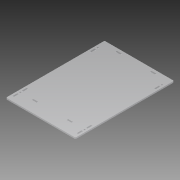
# Autodesk Inventor part: plastic_part_1
Saved by Autodesk Inventor 2013 (Build 170138000, 138)
## iProperties
Shininess: 20.0
Created: 2013-02-12
Part Number: plastic_part_1
Document SubType Name: Modeling
Designer: Noa Izumi
Material: Default
Density: 1 g/cm^3
Density: 0.0
Volumn: 0.0
Area: 0.0
PropertySet Name: Model Information
Control State: 0
Master: False
Checked Out: False
Author: Noa Izumi
Autodesk Inventor part; units mm, degrees
ref_plane "YZ Plane" through (0, 0, 0) normal (1, 0, 0) x (0, 1, 0)
ref_plane "XZ Plane" through (0, 0, 0) normal (0, 1, 0) x (-1, 0, 0)
ref_plane "XY Plane" through (0, 0, 0) normal (0, 0, 1) x (1, 0, 0)
sketch "Sketch1" plane through (0, 0, 0) normal (0, 0, 1) x (1, 0, 0)
  line L0 (0, 0) -> (148, 0)
  line L1 (148, 0) -> (148, 210)
  line L2 (148, 210) -> (0, 210)
  line L3 (0, 210) -> (0, 0)
  dimension "d0" = 148
  dimension "d1" = 210
  constraints: 8 end point, 2 parallel, 1 horizontal, 1 perpendicular
  measures "d0" distance of L0.start L0.end
  measures "d1" distance of L2.end L0.start
extrude "Extrusion1" add sketch "Sketch1" along normal blind 3
sketch "Sketch2" plane through (0, 0, 3) normal (0, 0, 1) x (1, 0, 0)
  line L0 (0, 0) -> (0, 210) projected
  line L1 (148, 0) -> (0, 0) projected
  line L2 (148, 210) -> (148, 0) projected
  line L3 (0, 210) -> (148, 210) projected
  line L4 (4, 185) -> (7, 185)
  line L5 (7, 185) -> (7, 175)
  line L6 (7, 175) -> (4, 175)
  line L7 (4, 175) -> (4, 185)
  line L8 (4, 40) -> (7, 40)
  line L9 (7, 40) -> (7, 30)
  line L10 (7, 30) -> (4, 30)
  line L11 (4, 30) -> (4, 40)
  line L12 (4, 20) -> (7, 20)
  line L13 (7, 20) -> (7, 10)
  line L14 (7, 10) -> (4, 10)
  line L15 (4, 10) -> (4, 20)
  line L16 (141, 175) -> (144, 175)
  line L17 (144, 175) -> (144, 185)
  line L18 (144, 185) -> (141, 185)
  line L19 (141, 185) -> (141, 175)
  line L20 (141, 40) -> (144, 40)
  line L21 (144, 40) -> (144, 30)
  line L22 (144, 30) -> (141, 30)
  line L23 (141, 30) -> (141, 40)
  line L24 (141, 20) -> (144, 20)
  line L25 (144, 20) -> (144, 10)
  line L26 (144, 10) -> (141, 10)
  line L27 (141, 10) -> (141, 20)
  dimension "d4" = 4
  dimension "d5" = 3
  dimension "d6" = 10
  dimension "d7" = 25
  dimension "d10" = 10
  dimension "d11" = 10
  dimension "d12" = 10
  dimension "d13" = 10
  dimension "d14" = 3
  dimension "d15" = 4
  dimension "d17" = 10
  dimension "d18" = 10
  dimension "d19" = 10
  dimension "d43" = 4
  dimension "d44" = 4
  dimension "d45" = 3
  dimension "d46" = 3
  dimension "d51" = 4
  dimension "d52" = 3
  dimension "d165" = 10
  dimension "d166" = 25
  dimension "d169" = 3
  constraints: 48 end point, 12 parallel, 6 horizontal, 6 perpendicular
  measures "d4" distance between parallel lines of L0 L7
  measures "d5" distance of L4.start L4.end
  measures "d6" distance of L6.end L4.start
  measures "d7" distance between parallel lines of L4 L3
  measures "d10" distance of L10.end L8.start
  measures "d11" distance between parallel lines of L12 L10
  measures "d12" distance of L14.end L12.start
  measures "d13" distance between parallel lines of L1 L14
  measures "d14" distance of L16.start L16.end
  measures "d15" distance between parallel lines of L2 L17
  measures "d17" distance of L20.end L21.end
  measures "d18" distance of L24.end L25.end
  measures "d19" distance between parallel lines of L24 L22
  measures "d43" distance between parallel lines of L2 L21
  measures "d44" distance between parallel lines of L2 L25
  measures "d45" distance of L20.start L20.end
  measures "d46" distance of L25.end L26.end
  measures "d51" distance between parallel lines of L0 L15
  measures "d52" distance of L9.end L10.end
  measures "d165" distance of L16.end L17.end
  measures "d166" distance between parallel lines of L18 L3
  measures "d169" distance of L13.end L14.end
extrude "Extrusion2" cut sketch "Sketch2" against normal through all contours L4 L5 L6 L7 | L8 L9 L10 L11 | L12 L13 L14 L15 | L19 L18 L17 L16 | L20 L21 L22 L23 | L24 L25 L26 L27
sketch "Sketch3" plane through (0, 0, 3) normal (0, 0, 1) x (1, 0, 0)
  line L0 (7, 30) -> (4, 30) projected
  line L1 (0, 210) -> (148, 210) projected
  line L2 (4, 175) -> (4, 185) projected
  line L3 (141, 175) -> (141, 185) projected
  line L4 (7, 40) -> (7, 30) projected
  point P0 (5.5, 190)
  point P1 (142.5, 190)
  point P2 (5.5, 25)
  point P3 (142.5, 25)
  point P4 (141, 30)
  dimension "d24" = 5
  dimension "d54" = 1.5
  dimension "d162" = 20
  dimension "d163" = 20
  dimension "d167" = 1.5
  dimension "d168" = 1.5
  dimension "d170" = 1.5
  measures "d24" distance from line of point (5.5, 25) L0
  measures "d54" horizontal distance of point (141, 30) point (142.5, 25)
  measures "d162" distance from line of L1 point (5.5, 190)
  measures "d163" distance from line of point (142.5, 190) L1
  measures "d167" distance from line of L2 point (5.5, 190)
  measures "d168" distance from line of L3 point (142.5, 190)
  measures "d170" distance from line of L4 point (5.5, 25)
hole "Hole1" at (5.5, 190, 3) at (142.5, 190, 3) at (5.5, 25, 3) at (142.5, 25, 3) direction (0, 0, -1) diameter 3 end through all
sketch "草圖12" plane through (0, 0, 3) normal (0, 0, 1) x (1, 0, 0)
  line L0 (0, 0) -> (0, 210) projected
  line L1 (148, 0) -> (0, 0) projected
  line L2 (148, 210) -> (148, 0) projected
  line L3 (0, 210) -> (148, 210) projected
  line L4 (32, 204.5) -> (42, 204.5)
  line L5 (42, 204.5) -> (42, 201.5)
  line L6 (42, 201.5) -> (32, 201.5)
  line L7 (32, 201.5) -> (32, 204.5)
  line L8 (106, 201.5) -> (116, 201.5)
  line L9 (116, 201.5) -> (116, 204.5)
  line L10 (116, 204.5) -> (106, 204.5)
  line L11 (106, 204.5) -> (106, 201.5)
  line L12 (32, 23.5) -> (42, 23.5)
  line L13 (42, 23.5) -> (42, 26.5)
  line L14 (42, 26.5) -> (32, 26.5)
  line L15 (32, 26.5) -> (32, 23.5)
  line L16 (106, 26.5) -> (116, 26.5)
  line L17 (116, 26.5) -> (116, 23.5)
  line L18 (116, 23.5) -> (106, 23.5)
  line L19 (106, 23.5) -> (106, 26.5)
  dimension "d148" = 3
  dimension "d150" = 10
  dimension "d151" = 32
  dimension "d152" = 5.5
  dimension "d153" = 10
  dimension "d154" = 32
  dimension "d155" = 3
  dimension "d156" = 23.5
  dimension "d157" = 32
  dimension "d158" = 32
  constraints: 32 end point, 8 parallel, 4 horizontal, 4 perpendicular
  measures "d148" distance of L4.end L5.end
  measures "d150" distance of L4.start L4.end
  measures "d151" distance between parallel lines of L7 L0
  measures "d152" distance between parallel lines of L4 L3
  measures "d153" distance of L9.end L10.end
  measures "d154" distance between parallel lines of L2 L9
  measures "d155" distance of L12.end L13.end
  measures "d156" distance between parallel lines of L1 L12
  measures "d157" distance between parallel lines of L2 L17
  measures "d158" distance between parallel lines of L0 L15
extrude "擠出5" cut sketch "草圖12" against normal through all contours L4 L5 L6 L7 | L11 L10 L9 L8 | L15 L14 L13 L12 | L16 L17 L18 L19
fillet "圓角3" radius 2 4 edges at (0, 0, 1.5) (148, 0, 1.5) (0, 210, 1.5) (148, 210, 1.5)
